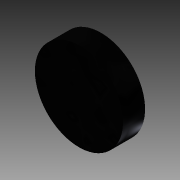
# Autodesk Inventor part: nóżka
Saved by Autodesk Inventor 2014 (Build 180170000, 170)
## iProperties
Created: 2013-08-20
Part Number: nóżka
Material: Tworzywo sztuczne SAN
Document SubType Name: Modeling
Designer: Kisieel
Density: 1 g/cm^3
Appearance: Czarny
Author: Kisieel
Autodesk Inventor part; units mm, degrees
ref_plane "YZ Plane" through (0, 0, 0) normal (1, 0, 0) x (0, 1, 0)
ref_plane "XZ Plane" through (0, 0, 0) normal (0, 1, 0) x (-1, 0, 0)
ref_plane "XY Plane" through (0, 0, 0) normal (0, 0, 1) x (1, 0, 0)
sketch "Szkic1" plane through (0, 0, 0) normal (0, 1, 0) x (-1, 0, 0)
  circle A0 centre (0, 0) radius 10
  dimension "d0" = 20
  constraints: 1 centre point, 1 coincident
  measures "d0" diameter of A0
extrude "Wyciągnięcie proste1" add sketch "Szkic1" along normal blind 5
